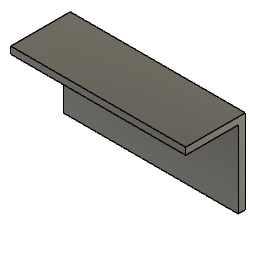
soap holder bracket part 2 v4 (Autodesk Fusion 360 design; units mm, degrees)
Autodesk Fusion 360 part; units mm, degrees
sketch "Sketch1" plane through (0, 0, 0) normal (0, 1, 0) x (1, 0, 0)
  line L0 (0, 0) -> (50, 0)
  line L1 (50, 0) -> (50, -24)
  line L2 (50, -24) -> (0, -24)
  line L3 (0, -24) -> (0, 0)
  constraint horizontal L0
  constraint vertical L1
  constraint horizontal L2
  constraint vertical L3
  constraint coincident L0.start L3.end
extrude "Extrude1" add sketch "Sketch1" along normal blind 2
sketch "Sketch2" plane through (0, 0, 0) normal (0, 1, 0) x (1, 0, 0)
  line L0 (0, -24) -> (50, -24)
  line L1 (50, -24) -> (50, -22)
  line L2 (50, -22) -> (0, -22)
  line L3 (0, -22) -> (0, -24)
  constraint horizontal L0
  constraint vertical L1
  constraint horizontal L2
  constraint vertical L3
extrude "Extrude2" add sketch "Sketch2" against normal blind 15
sketch "Sketch3" plane through (0, 0, 0) normal (0, 1, 0) x (1, 0, 0)
  line L0 (17, -20) -> (19, -20)
  line L1 (19, -20) -> (19, -8)
  line L2 (19, -8) -> (17, -8)
  line L3 (17, -8) -> (17, -20)
  constraint horizontal L0
  constraint vertical L1
  constraint horizontal L2
  constraint vertical L3
extrude "Extrude3" cut sketch "Sketch3" along normal blind 5
sketch "Sketch4" plane through (0, 0, 0) normal (0, 1, 0) x (1, 0, 0)
  line L0 (33, -20) -> (31, -20)
  line L1 (31, -20) -> (31, -8)
  line L2 (31, -8) -> (33, -8)
  line L3 (33, -8) -> (33, -20)
  constraint horizontal L0
  constraint vertical L1
  constraint horizontal L2
  constraint vertical L3
extrude "Extrude4" cut sketch "Sketch4" along normal blind 3
